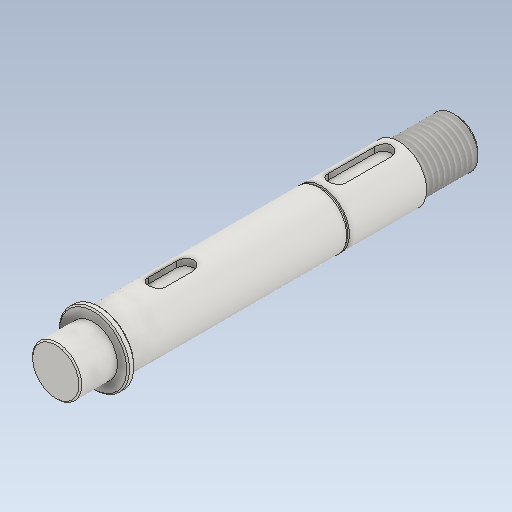
# Autodesk Inventor part: Peça12
Saved by Autodesk Inventor 2021 (Build 250183000, 183)
## iProperties
Category: 42
Created: 2021-07-17
Part Number: Peça12
Material: Liga de aço
Document SubType Name: Modeling
Designer: Giovanni
Density: 7.73 g/cm^3
Appearance: Aço
User Status: 1:3
Author: Giovanni
Keywords: 9
Autodesk Inventor part; units mm, degrees
ref_plane "YZ Plane" through (0, 0, 0) normal (1, 0, 0) x (0, 1, 0)
ref_plane "XY Plane" through (0, 0, 0) normal (0, 0, 1) x (1, 0, 0)
sketch "Esboço1" plane through (0, 0, 0) normal (0, 0, 1) x (-1, 0, 0)
  circle A0 centre (0, 0) radius 25
  dimension "d0" = 50
  constraints: 1 centre point, 1 coincident
  measures "d0" diameter of A0
extrude "Extrusão1" add sketch "Esboço1" along normal mid plane 5
sketch "Esboço2" plane through (0, 0, 0) normal (0, 0, -1) x (1, 0, 0)
  circle A0 centre (0, 0) radius 20
  dimension "d3" = 40
  constraints: 1 centre point, 1 coincident
  measures "d3" diameter of A0
extrude "Extrusão2" add sketch "Esboço2" along normal blind 215
sketch "Esboço3" plane through (0, 0, 0) normal (0, 0, 1) x (1, 0, 0)
  circle A0 centre (0, 0) radius 17.5
  dimension "d6" = 35
  constraints: 1 centre point, 1 coincident
  measures "d6" diameter of A0
extrude "Extrusão3" add sketch "Esboço3" along normal blind 29
chamfer "Chanfro2" distance 1 angle 45 3 edges at (25, 0, -2.5) (25, 0, 2.5) (-17.5, 0, 29)
ref_plane "Plano de trabalho2" through (0, 20, 0) normal (0, 1, 0) x (-1, 0, 0)
sketch "Esboço7" plane through (0, 20, 0) normal (0, 1, 0) x (-1, 0, 0)
  line L0 (0, -63) -> (0, -43) construction
  line L1 (6, -63) -> (6, -43)
  line L2 (-6, -43) -> (-6, -63)
  arc A0 (-6, -63) -> (6, -63) centre (0, -63) ccw
  arc A1 (6, -43) -> (-6, -43) centre (0, -43) ccw
  line L3 (24, -2.5) -> (-24, -2.5) projected
  point P0 (0, 0)
  point P1 (0, -53)
  dimension "d25" = 12
  dimension "d26" = 20
  dimension "d27" = 40.5
  constraints: 8 end point, 4 point on circle, 4 tangent, 2 centre point, 1 midpoint, 1 parallel, 1 vertical
  measures "d25" diameter of A1
  measures "d26" distance of L0.start L0.end
  measures "d27" distance from line of L3 L0.end
extrude "Extrusão6" cut sketch "Esboço7" against normal blind 5
sketch "Esboço8" plane through (0, 0, -215) normal (0, 0, -1) x (-1, 0, 0)
  circle A0 centre (0, 0) radius 20 projected
  circle A1 centre (0, 0) radius 17.5
  dimension "d30" = 35
  constraints: 1 centre point, 1 coincident
  measures "d30" diameter of A1
extrude "Extrusão7" add sketch "Esboço8" along normal blind 3 contours A1
sketch "Esboço9" plane through (0, 0, -218) normal (0, 0, -1) x (-1, 0, 0)
  circle A0 centre (0, 0) radius 17.5 projected
  circle A1 centre (0, 0) radius 19.5
  dimension "d33" = 39
  constraints: 1 centre point, 1 coincident
  measures "d33" diameter of A1
extrude "Extrusão8" add sketch "Esboço9" along normal blind 38 contours A0
chamfer "Chanfro3" distance 2 angle 45 1 edges at (17.5, 0, -256)
thread "Rosca1" size "M39x4" class "6g" standard "ANSI Metric M Profile" full length
sketch "Esboço10" plane through (0, 0, 0) normal (1, 0, 0) x (0, 1, 0)
  line L0 (20, -2.5) -> (20, -215) projected
  line L1 (20, -160) -> (18.75, -160)
  line L2 (18.75, -160) -> (18.75, -158.15)
  line L3 (18.75, -158.15) -> (20, -158.15)
  line L4 (20, -158.15) -> (20, -160)
  line L5 (0, 0) -> (0, -179.7731)
  dimension "d41" = 1.85
  dimension "d42" = 160
  dimension "d43" = 37.5
  constraints: 10 end point, 2 parallel, 1 horizontal, 1 perpendicular, 1 point on line, 1 vertical
  measures "d41" distance between parallel lines of L3 L1
  measures "d42" distance from line of L5.start L1
  measures "d43" diameter of L2 L5
revolve "Revolução1" cut sketch "Esboço10" angle 360 about axis through (0, 0, 0) along (0, 0, -1)
sketch "Esboço11" plane through (0, 20, 0) normal (0, 1, 0) x (-1, 0, 0)
  line L0 (0, -204) -> (0, -171) construction
  line L1 (6, -204) -> (6, -171)
  line L2 (-6, -171) -> (-6, -204)
  arc A0 (-6, -204) -> (6, -204) centre (0, -204) ccw
  arc A1 (6, -171) -> (-6, -171) centre (0, -171) ccw
  point P0 (0, 0)
  point P1 (0, -187.5)
  dimension "d45" = 171
  dimension "d46" = 33
  dimension "d47" = 6
  constraints: 8 end point, 4 point on circle, 4 tangent, 2 centre point, 1 midpoint, 1 parallel, 1 vertical, 1 vertical alignment
  measures "d45" distance of point (0, 0) L0.end
  measures "d46" distance of L0.end L0.start
  measures "d47" radius of A0
extrude "Extrusão9" cut sketch "Esboço11" against normal blind 5
